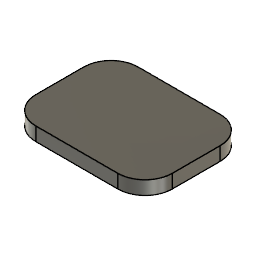
day-21-one-part-molds (Autodesk Fusion 360 design; units mm, degrees)
part number: 2026-06-15-17-20-42-627
part number: 2026-06-15-19-28-05-085
part number: 2026-06-15-19-33-53-219
Autodesk Fusion 360 part; units mm, degrees
sketch "Sketch1" plane through (0, 0, 0) normal (0, 0, 1) x (1, 0, 0) in component "Keychain"
  line L0 (0, 0) -> (50, 0)
  line L1 (50, 0) -> (50, -35)
  line L2 (50, -35) -> (0, -35)
  line L3 (0, -35) -> (0, 0)
  dimension "d1" = 50
  dimension "d2" = 35
  constraint horizontal L0
  constraint vertical L1
  constraint horizontal L2
  constraint vertical L3
  constraint coincident L0.start L3.end
  measures "d1" distance of L0.start L0.end
  measures "d2" distance of L0.start L2.end
extrude "Extrude1" add sketch "Sketch1" along normal blind 3 makes body 1 in component "Keychain"
fillet "Fillet1" radius 7 4 edges at (50, -35, 1.5) (0, -35, 1.5) (0, 0, 1.5) (50, 0, 1.5) on bodies 1 in component "Keychain"
sketch "Sketch2" plane through (0, 0, 3) normal (0, 0, 1) x (-1, 0, 0) in component "Keychain"
  arc A0 (-50, 7) -> (-43, 0) centre (-43, 7) ccw
  line L0 (-43, 0) -> (-7, 0)
  arc A1 (-7, 0) -> (0, 7) centre (-7, 7) ccw
  line L1 (0, 7) -> (0, 28)
  arc A2 (0, 28) -> (-7, 35) centre (-7, 28) ccw
  line L2 (-7, 35) -> (-43, 35)
  arc A3 (-43, 35) -> (-50, 28) centre (-43, 28) ccw
  line L3 (-50, 28) -> (-50, 7)
  line L4 (-50, 17.5) -> (-45, 17.5) construction
  dimension "d7" = 5
  constraint midpoint L3 L4.start
  constraint perpendicular L3 L4
  measures "d7" distance of L4.start L4.end
hole "Hole1" at (45, -17.5, 3) direction (0, 0, -1) diameter 5 end up to surface (3 mm away) bodies 1 in component "Keychain"
sketch "Sketch3" plane through (0, 0, 3) normal (0, 0, 1) x (-1, 0, 0) in component "Keychain"
  circle A0 centre (-45, 17.5) radius 2.5
  arc A1 (-50, 7) -> (-43, 0) centre (-43, 7) ccw
  line L0 (-43, 0) -> (-7, 0)
  arc A2 (-7, 0) -> (0, 7) centre (-7, 7) ccw
  line L1 (0, 7) -> (0, 28)
  arc A3 (0, 28) -> (-7, 35) centre (-7, 28) ccw
  line L2 (-7, 35) -> (-43, 35)
  arc A4 (-43, 35) -> (-50, 28) centre (-43, 28) ccw
  line L3 (-50, 28) -> (-50, 7)
  line L4 (0, 35) -> (-42, 35) construction
  line L5 (-42, 35) -> (-42, 0) construction
  line L6 (-42, 0) -> (0, 0) construction
  line L7 (0, 0) -> (0, 35) construction
  dimension "d10" = 8
  text T0 "Ekansh" font "Arial" height 8 bold align centre middle in box 42 x 35 at (0, 35) x (-1, 0) y (0, -1) spacing 1 kerned
  constraint coincident L2
  constraint coincident L6.end
extrude "Extrude2" add sketch "Sketch3" along normal blind 2 text T0 bodies 1 in component "Keychain"
sketch "Sketch1 (2)" plane through (0, 0, 0) normal (0, 0, 1) x (1, 0, 0) in component "One-Part-Mold"
  circle A0 centre (45, -17.5) radius 2.5
  arc A1 (50, -7) -> (43, 0) centre (43, -7) ccw
  line L0 (7, 0) -> (43, 0)
  arc A2 (7, 0) -> (0, -7) centre (7, -7) ccw
  line L1 (0, -28) -> (0, -7)
  arc A3 (0, -28) -> (7, -35) centre (7, -28) ccw
  line L2 (43, -35) -> (7, -35)
  arc A4 (43, -35) -> (50, -28) centre (43, -28) ccw
  line L3 (50, -7) -> (50, -28)
  arc A5 (55, -7) -> (43, 5) centre (43, -7) ccw
  line L4 (7, 5) -> (43, 5)
  arc A6 (7, 5) -> (-5, -7) centre (7, -7) ccw
  line L5 (-5, -28) -> (-5, -7)
  arc A7 (-5, -28) -> (7, -40) centre (7, -28) ccw
  line L6 (43, -40) -> (7, -40)
  arc A8 (43, -40) -> (55, -28) centre (43, -28) ccw
  line L7 (55, -7) -> (55, -28)
  dimension "d14" = -5
extrude "Extrude1'" add sketch "Sketch1 (2)" along normal blind 6 separate body contours A0 | A1 L0 A2 L1 A3 L2 A4 L3 | A5 L4 A6 L5 A7 L6 A8 L7 makes body 2 in component "One-Part-Mold"
combine "Combine1" operation cut target body 2 tool bodies 1 keep tools in component "One-Part-Mold"
draft "Draft1" angle 5 neutral plane through (0, 0, 0) pull (0, 0, -1) 9 faces at (19, 0, 2) (49.9921, -6.6669, 1) (50, -14, 1) (43.3331, -34.9921, 1) (31, -35, 1) (1.298, -32.0604, 1) (0, -21, 1) (0.0079, -6.6669, 1) (45.1246, -19.9969, 2) on bodies 2 in component "One-Part-Mold"
component "Keychain" placed x (1, 0, 0) y (0, 1, 0) z (0, 0, 1) at (0, 0, 0)
component "One-Part-Mold" placed x (1, 0, 0) y (0, 1, 0) z (0, 0, 1) at (0, 0, 0)
hidden bodies 1
equation "d11 = 'Ekansh'"
